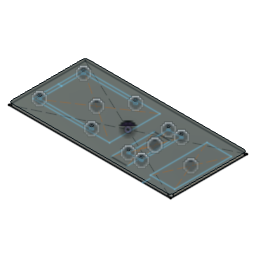
_pcb-footprint.d29b2546-1c5a-49bb-88ae-6fe5814387b5 (Autodesk Fusion 360 design; units mm, degrees)
Autodesk Fusion 360 part; units mm, degrees
sketch "Sketch1" plane through (0, 0, 0) normal (0, 0, 1) x (1, 0, 0)
  line L0 (90, 42.5) -> (-90, 42.5)
  line L1 (-90, 42.5) -> (-90, -42.5)
  line L2 (-90, -42.5) -> (90, -42.5)
  line L3 (90, -42.5) -> (90, 42.5)
  line L4 (90, 42.5) -> (-90, -42.5) construction
  line L5 (-90, 42.5) -> (90, -42.5) construction
  line L6 (2.5, 33) -> (-82.5, 33)
  line L7 (-82.5, 33) -> (-82.5, -23)
  line L8 (-82.5, -23) -> (2.5, -23)
  line L9 (2.5, -23) -> (2.5, 33)
  line L10 (2.5, 33) -> (-82.5, -23) construction
  line L11 (-82.5, 33) -> (2.5, -23) construction
  line L12 (-82.5, 5) -> (-79, 5)
  line L13 (-79, 5) -> (-79, 29.5)
  line L14 (-79, 5) -> (-79, -19.5)
  line L15 (-79, -19.5) -> (-21, -19.5)
  line L16 (-79, 29.5) -> (-21, 29.5)
  circle A0 centre (-79, -19.5) radius 1.5
  circle A1 centre (-79, 29.5) radius 1.5
  circle A2 centre (-21, 29.5) radius 1.5
  circle A3 centre (-21, -19.5) radius 1.5
  line L17 (16.6875, -35.5) -> (34.6875, -35.5)
  line L18 (34.6875, -35.5) -> (34.6875, 12.5)
  line L19 (34.6875, 12.5) -> (16.6875, 12.5)
  line L20 (16.6875, 12.5) -> (16.6875, -35.5)
  line L21 (16.6875, -35.5) -> (34.6875, 12.5) construction
  line L22 (34.6875, -35.5) -> (16.6875, 12.5) construction
  line L23 (37.25, 22.25) -> (22.75, 22.25)
  line L24 (22.75, 22.25) -> (22.75, -22.25)
  line L25 (22.75, -22.25) -> (37.25, -22.25)
  line L26 (37.25, -22.25) -> (37.25, 22.25)
  line L27 (37.25, 22.25) -> (22.75, -22.25) construction
  line L28 (22.75, 22.25) -> (37.25, -22.25) construction
  circle A4 centre (22.75, 22.25) radius 1.25
  circle A5 centre (37.25, 22.25) radius 1.25
  circle A6 centre (37.25, -22.25) radius 1.25
  circle A7 centre (22.75, -22.25) radius 1.25
  line L29 (59.5276, -35.5) -> (59.5276, -42.5)
  line L30 (83.5, 31.5) -> (56.5, 31.5)
  line L31 (56.5, 31.5) -> (56.5, -31.5)
  line L32 (56.5, -31.5) -> (83.5, -31.5)
  line L33 (83.5, -31.5) -> (83.5, 31.5)
  line L34 (83.5, 31.5) -> (56.5, -31.5) construction
  line L35 (56.5, 31.5) -> (83.5, -31.5) construction
  point P0 (-40, 5)
  point P1 (30, 0)
  point P2 (30, 0)
  point P3 (70, 0)
  dimension "d1" = 180
  dimension "d2" = 85
  dimension "d3" = 85
  dimension "d4" = 56
  dimension "d5" = 3.5
  dimension "d6" = 24.5
  dimension "d7" = 24.5
  dimension "d8" = 58
  dimension "d9" = 58
  dimension "d10" = 3
  dimension "d11" = 3
  dimension "d12" = 3
  dimension "d13" = 3
  dimension "d16" = 18
  dimension "d17" = 48
  dimension "d18" = 14.5
  dimension "d19" = 44.5
  dimension "d20" = 2.5
  dimension "d21" = 2.5
  dimension "d22" = 2.5
  dimension "d23" = 2.5
  dimension "d26" = 7
  dimension "d29" = 27
  dimension "d30" = 63
  constraint horizontal L0
  constraint perpendicular L0 L1
  constraint parallel L0 L2
  constraint parallel L1 L3
  constraint coincident L4 origin
  constraint coincident L5 origin
  constraint horizontal L6
  constraint perpendicular L6 L7
  constraint parallel L6 L8
  constraint parallel L7 L9
  constraint coincident L10 P0
  constraint coincident L11 P0
  constraint midpoint L7 L12.start
  constraint perpendicular L7 L12
  constraint perpendicular L12 L13
  constraint perpendicular L12 L14
  constraint perpendicular L14 L15
  constraint perpendicular L13 L16
  constraint coincident L14.end L15.start
  constraint coincident L13.end L16.start
  constraint coincident L16.end A2.centre
  constraint coincident L15.end A3.centre
  constraint horizontal L17
  constraint perpendicular L17 L18
  constraint parallel L17 L19
  constraint parallel L18 L20
  constraint coincident L21 P2
  constraint horizontal L23
  constraint perpendicular L23 L24
  constraint parallel L23 L25
  constraint parallel L24 L26
  constraint coincident L27 P2
  constraint coincident L28 P2
  constraint coincident P2 P1
  constraint coincident L23.end L24.start
  constraint coincident L23.start L26.end
  constraint coincident L25.end L26.start
  constraint coincident L24.end L25.start
  constraint coincident L17 L29.start
  constraint coincident L2 L29.end
  constraint perpendicular L2 L29
  constraint horizontal L30
  constraint perpendicular L30 L31
  constraint parallel L30 L32
  constraint parallel L31 L33
  constraint coincident L34 P3
  constraint coincident L35 P3
  measures "d1" distance of L1 L3
  measures "d2" distance of L0.end L1.end
  measures "d3" distance of L7.end L8.end
  measures "d4" distance of L6.end L7.end
  measures "d5" distance of L12.start L12.end
  measures "d6" distance of L12.end L13.end
  measures "d7" distance of L12.end L14.end
  measures "d8" distance of L14.end L15.end
  measures "d9" distance of L13.end L16.end
  measures "d10" diameter of A0
  measures "d11" diameter of A1
  measures "d12" diameter of A2
  measures "d13" diameter of A3
  measures "d16" distance of L18.end L19.end
  measures "d17" distance of L17.end L18.end
  measures "d18" distance of L24.end L25.end
  measures "d19" distance of L23.end L24.end
  measures "d20" diameter of A4
  measures "d21" diameter of A5
  measures "d22" diameter of A6
  measures "d23" diameter of A7
  measures "d26" distance of L29.start L29.end
  measures "d29" distance of L31.end L32.end
  measures "d30" distance of L30.end L31.end
extrude "Extrude2" add sketch "Sketch1" along normal blind 3 contours L0 L1 L2 L3 | L6 L7 L8 L9 | L17 L18 L19 L20 L24 L25 A7 | L18 L19 L24 L25 A7 | L18 L19 L23 L24 L25 L26 A4 A5 A6 | L30 L31 L32 L33
fillet "Fillet1" radius 3 4 edges at (-90, 42.5, 1.5) (-90, -42.5, 1.5) (90, 42.5, 1.5) (90, -42.5, 1.5)
sketch "Sketch5" plane through (0, 0, 3) normal (0, 0, 1) x (-1, 0, 0)
  arc A0 (-87, 42.5) -> (-90, 39.5) centre (-87, 39.5) ccw
  line L0 (-90, 39.5) -> (-90, -39.5)
  arc A1 (-90, -39.5) -> (-87, -42.5) centre (-87, -39.5) ccw
  line L1 (-87, -42.5) -> (87, -42.5)
  arc A2 (87, -42.5) -> (90, -39.5) centre (87, -39.5) ccw
  line L2 (90, -39.5) -> (90, 39.5)
  arc A3 (90, 39.5) -> (87, 42.5) centre (87, 39.5) ccw
  line L3 (87, 42.5) -> (-87, 42.5)
  circle A4 centre (79, -29.5) radius 1.5
  circle A5 centre (79, 19.5) radius 1.5
  circle A6 centre (21, -29.5) radius 1.5
  circle A7 centre (-22.75, 22.25) radius 1.25
  circle A8 centre (-37.25, 22.25) radius 1.25
  circle A9 centre (-37.25, -22.25) radius 1.25
  circle A10 centre (-22.75, -22.25) radius 1.25
  circle A11 centre (21, 19.5) radius 1.5
equation "d18 = 18 mm - 3.5 mm"
equation "d19 = 48 mm - 3.5 mm"
